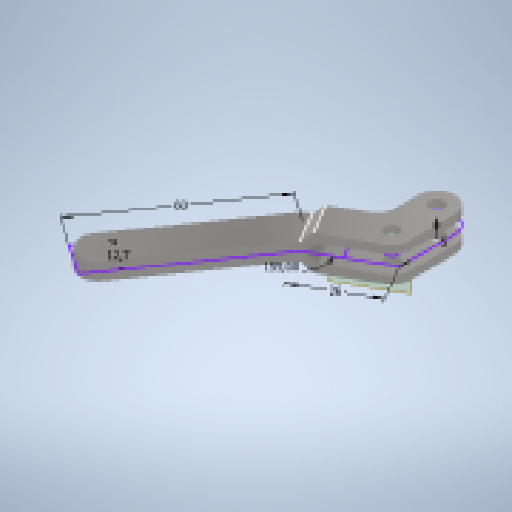
# Autodesk Inventor part: part2
Saved by Autodesk Inventor 2025.2 (Build 292293000, 293)
## iProperties
Created: 2024-12-06
Part Number: part2
Material: Stal nierdzewna
Document SubType Name: Modeling
Designer: Marek
Density: 8 g/cm^3
Appearance: Częściowo polerowany
Author: Marek
Autodesk Inventor part; units mm, degrees
ref_plane "YZ Plane" through (0, 0, 0) normal (1, 0, 0) x (0, 1, 0)
ref_plane "XZ Plane" through (0, 0, 0) normal (0, 1, 0) x (-1, 0, 0)
ref_plane "XY Plane" through (0, 0, 0) normal (0, 0, 1) x (1, 0, 0)
sketch "Szkic1" plane through (0, 0, 0) normal (0, 1, 0) x (-1, 0, 0)
  line L0 (12.7, -3.666174) -> (12.7, -16)
  line L1 (0, -16) -> (0, 0)
  arc A0 (0, -16) -> (12.7, -16) centre (6.35, -16) ccw
  line L2 (0, 3.666174) -> (22.51666, 16.666174)
  line L3 (0, 0) -> (0, 3.666174)
  line L4 (22.51666, 16.666174) -> (55.316329, 63.508956)
  line L5 (65.71956, 56.224535) -> (31.304974, 7.075413)
  circle A1 centre (6.35, -16) radius 2.5
  circle A2 centre (6.35, 0) radius 2.5
  line L6 (65.71956, 56.224535) -> (55.316329, 63.508956)
  line L7 (22.51666, 16.666174) -> (28.86666, 5.667652)
  line L8 (31.304974, 7.075413) -> (12.7, -3.666174)
  line L9 (19.05, 0) -> (12.7, 10.998523)
  dimension "d5" = 155
  dimension "d7" = 5
  dimension "d9" = 26
  dimension "d11" = 12.7
  dimension "d13" = 60
  constraints: 20 end point, 3 centre point, 3 point on line, 2 point on circle, 1 coincident, 1 equal radius, 1 parallel, 1 perpendicular, 1 vertical
  measures "d5" angle of L2 L4
  measures "d7" diameter of A1
  measures "d9" distance of L2.start L2.end
  measures "d11" distance between parallel lines of L4 L5
  measures "d13" distance of L5.start L5.end
extrude "Wyciągnięcie proste1" add sketch "Szkic1" against normal blind 3 contours L7 L4 L6 L5 L8
ref_plane "Płaszczyzna konstrukcyjna1" through (-15.875, -6.175, -1.833087) normal (-0.5, 0, -0.8660254) x (-0.8660254, 0, 0.5)
sketch "Szkic2" plane through (-15.875, -6.175, -1.833087) normal (-0.5, 0, -0.8660254) x (-0.8660254, 0, 0.5)
  line L0 (15.001477, 3.175) -> (11.826477, 0)
  line L1 (11.799797, -0.02668) -> (15.001477, 3.175)
  line L2 (12.880157, 5.29632) -> (10.583837, 3)
  line L3 (15.001477, 3.175) -> (15.001477, 6.175)
  line L4 (0, 6.175) -> (16.409238, 6.175)
  line L5 (12.880157, 5.29632) -> (13.758837, 6.175)
  line L6 (15.001477, 3.175) -> (11.826477, 0)
  line L7 (13.758837, 6.175) -> (15.001477, 6.175)
  line L8 (15.001477, 6.175) -> (15.001477, 3.175)
  line L9 (10.583837, 3) -> (0, 3)
  line L10 (10.583837, 3) -> (10.583837, 3)
  line L11 (0, 3) -> (0, 0)
  line L12 (0, 0) -> (11.826477, 0)
  line L13 (11.826477, 0) -> (11.826477, 0)
  point P0 (-12.83161, 6.175)
  dimension "d27" = 3
  dimension "d34" = 3.175
  constraints: 22 end point, 3 point on line, 2 collinear, 2 perpendicular, 2 vertical, 1 horizontal
  measures "d27" distance of L9.end L11.end
  measures "d34" distance between parallel lines of L4 L9
extrude "Wyciągnięcie proste3" add sketch "Szkic2" against normal blind 12.7
extrude "Wyciągnięcie proste4" add sketch "Szkic1" against normal blind 6.175 contours L0 A0 L1 L3 L2 L9 L8
extrude "Wyciągnięcie proste5" cut sketch "Szkic1" against normal blind 3.175 contours L0 A0 L1 L3 L2 L9 L8
fillet "Zaokrąglenie2" radius 1.5 4 edges at (-24.6155, 0, 10.5456) (-21.8659, -3.175, 8.9581) (-22.942, -6.175, 9.5794) (-25.6917, -3, 11.1669)
fillet "Zaokrąglenie3" radius 6.35 6 edges at (-12.7, -4.675, -3.6662) (-31.305, -1.5, 7.0754) (-65.7196, -1.5, 56.2245) (-22.5167, -1.5674, 16.6662) (0, -4.675, 3.6662) (-55.3163, -1.5, 63.509)
mirror "Odbij1" about plane through (-44.11811, 0, 34.588304) normal (0, 1, 0)
